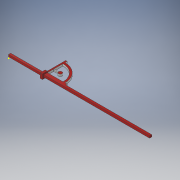
# Autodesk Inventor part: MiddleStick
Saved by Autodesk Inventor 2018.2 (Build 222227000, 227)
## iProperties
Created: 2018-04-10
Part Number: MiddleStick
Material: Generisch
Document SubType Name: Modeling
Designer: Nick Koch
Density: 1 g/cm^3
Appearance: Vorgabe
Author: Nick Koch
Autodesk Inventor part; units mm, degrees
ref_plane "YZ Plane" through (0, 0, 0) normal (1, 0, 0) x (0, 1, 0)
ref_plane "XZ Plane" through (0, 0, 0) normal (0, 1, 0) x (-1, 0, 0)
ref_plane "XY Plane" through (0, 0, 0) normal (0, 0, 1) x (1, 0, 0)
sketch "Skizze4" plane through (0, 0, 0) normal (0, 0, 1) x (1, 0, 0)
  line L0 (0, 0) -> (200, 0)
  line L1 (200, 0) -> (200, 3)
  line L2 (200, 3) -> (0, 3)
  line L3 (0, 3) -> (0, 0)
  dimension "d12" = 200
  dimension "d13" = 3
  constraints: 8 end point, 2 parallel, 1 horizontal, 1 perpendicular
  measures "d12" distance of L2.end L1.end
  measures "d13" distance of L1.end L0.end
extrude "Extrusion4" add sketch "Skizze4" along normal blind 3
sketch "Skizze5" plane through (0, 0, 3) normal (0, 0, 1) x (1, 0, 0)
  line L0 (47, 5) -> (50, 5)
  line L1 (50, 5) -> (50, -2)
  line L2 (50, -2) -> (47, -2)
  line L3 (47, -2) -> (47, 5)
  line L4 (200, 0) -> (200, 3) projected
  line L5 (0, 3) -> (0, 0) projected
  line L6 (200, 3) -> (0, 3) projected
  line L7 (0, 0) -> (200, 0) projected
  dimension "d16" = 150
  dimension "d17" = 47
  dimension "d18" = 2
  dimension "d19" = 2
  constraints: 8 end point, 2 parallel, 1 horizontal, 1 perpendicular
  measures "d16" distance between parallel lines of L4 L1
  measures "d17" distance between parallel lines of L5 L3
  measures "d18" distance between parallel lines of L0 L6
  measures "d19" distance between parallel lines of L7 L2
extrude "Extrusion5" add sketch "Skizze5" along normal blind 2 and the other way blind 5 contours L0 L1 L6 L3 | L6 L1 L7 L3 | L7 L1 L2 L3
sketch "Skizze6" plane through (0, 0, -2) normal (0, 0, -1) x (-1, 0, 0)
  point P0 (0, 0)
sketch "Skizze7" plane through (0, 0, 0) normal (0, 0, -1) x (-1, 0, 0)
  line L0 (-200, 3) -> (-50, 3) projected
  line L1 (-78, 3) -> (-50, 3)
  line L2 (-50, 3) -> (-50, 5)
  line L3 (-50, 5) -> (-78, 5)
  line L4 (-78, 5) -> (-78, 3)
  line L5 (-50, 5) -> (-48, 5)
  line L6 (-48, 5) -> (-48, 33)
  line L7 (-48, 33) -> (-50, 33)
  line L8 (-50, 33) -> (-50, 5)
  line L9 (-50, -2) -> (-50, 5) projected
  arc A0 (-50, 30) -> (-75, 5) centre (-50, 5) ccw
  arc A1 (-50, 27.2) -> (-72.2, 5) centre (-50, 5) ccw
  line L10 (-50, 5) -> (-59.1924, 14.1924)
  line L11 (-50, 5) -> (-37, 5) construction
  circle A2 centre (-59.1924, 14.1924) radius 2.5
  line L12 (-59.1924, 14.1924) -> (-50, 14.1924)
  line L13 (-59.1924, 14.1924) -> (-50, 14.1924)
  line L14 (-50, 14.1924) -> (-50, 13.3924)
  line L15 (-50, 13.3924) -> (-59.1924, 13.3924)
  line L16 (-59.1924, 13.3924) -> (-59.1924, 14.1924)
  line L17 (-50, 14.1924) -> (-59.1924, 14.1924)
  line L18 (-59.1924, 14.1924) -> (-59.1924, 14.9924)
  line L19 (-59.1924, 14.9924) -> (-50, 14.9924)
  line L20 (-50, 14.9924) -> (-50, 14.1924)
  line L21 (-50, 30) -> (-50, 27.2)
  line L22 (-75, 5) -> (-72.2, 5)
  point P0 (0, 0)
  dimension "d24" = 2
  dimension "d25" = 2
  dimension "d26" = 50
  dimension "d27" = 2.8
  dimension "d28" = 13
  dimension "d29" = 135
  dimension "d30" = 5
  dimension "d31" = 0.8
  dimension "d32" = 0.8
  dimension "d33" = 28
  dimension "d34" = 28
  constraints: 42 end point, 8 parallel, 7 perpendicular, 4 point on circle, 4 point on line, 3 centre point, 3 horizontal, 2 coincident, 1 collinear, 1 equal length, 1 vertical
  measures "d24" distance of L2.end L1.end
  measures "d25" distance of L7.end L6.end
  measures "d26" diameter of A0
  measures "d27" radial gap between concentric circles of A0 A1
  measures "d28" distance of L10.start L10.end
  measures "d29" angle of L11 L10
  measures "d30" diameter of A2
  measures "d31" distance of L12.end L14.end
  measures "d32" distance of L12.start L18.end
  measures "d33" distance of L5.end L6.end
  measures "d34" distance of L2.end L3.end
extrude "Extrusion6" add sketch "Skizze7" against normal blind 3 contours L4 L3 L2 L0 | L8 L7 L6 L5 | A0 L8 A1 L3 | L15 A2 L12 L8 | A2 L19 L18 L16 L15 L10 | L10 L15 A2 | L12 A2 L19 L8 | L15 L10 L12 A2 | L15 L16 L10 | A2 L12 L18 L19
sketch "Skizze8" plane through (0, 0, 0) normal (0, 0, -1) x (-1, 0, 0)
  arc A0 (-56.8238, 14.9924) -> (-56.8238, 13.3924) centre (-59.1924, 14.1924) ccw projected
  circle A1 centre (-59.1924, 14.1924) radius 2.5
  line L0 (-56.8238, 13.3924) -> (-50, 13.3924) projected
  line L1 (-56.8238, 13.3924) -> (-50, 13.3924)
  line L2 (-50, 13.3924) -> (-50, 14.9924)
  line L3 (-56.8238, 14.9924) -> (-50, 14.9924) projected
  line L4 (-50, 14.9924) -> (-56.8238, 14.9924)
  point P0 (0, 0)
  constraints: 6 end point, 2 perpendicular, 1 centre point, 1 coincident, 1 collinear
extrude "Extrusion7" cut sketch "Skizze8" against normal blind 0.75 contours L3 L2 L0 A1
sketch "Skizze9" plane through (0, 0, 3) normal (0, 0, 1) x (1, 0, 0)
  arc A0 (56.8238, 13.3924) -> (56.8238, 14.9924) centre (59.1924, 14.1924) ccw projected
  circle A1 centre (59.1924, 14.1924) radius 2.5
  line L0 (50, 14.9924) -> (50, 27.2) projected
  line L1 (56.8238, 14.9924) -> (50, 14.9924)
  line L2 (50, 14.9924) -> (50, 13.3924) projected
  line L3 (50, 14.9924) -> (50, 13.3924)
  line L4 (50, 13.3924) -> (56.8238, 13.3924)
  point P0 (0, 0)
  constraints: 6 end point, 2 perpendicular, 1 coincident, 1 horizontal, 3 other
extrude "Extrusion8" cut sketch "Skizze9" against normal blind 0.75 contours L4 L2 L1 A1
